Autodesk Fusion 360 part; units mm, degrees
(part 3 of 3)
  constraint equal A304 A396
  constraint tangent L88 A397
  constraint tangent L89 A397
  constraint equal A304 A397
  constraint tangent L88 A398
  constraint tangent L90 A398
  constraint equal A304 A398
  constraint tangent L90 A399
  constraint tangent L91 A399
  constraint equal A304 A399
  constraint tangent L93 A400
  constraint tangent L95 A400
  constraint equal A304 A400
  constraint tangent L92 A401
  constraint tangent L93 A401
  constraint equal A304 A401
  constraint tangent L92 A402
  constraint tangent L94 A402
  constraint equal A304 A402
  constraint tangent L94 A403
  constraint tangent L95 A403
  constraint equal A304 A403
  constraint tangent L120 A404
  constraint tangent L121 A404
  constraint equal A304 A404
  constraint tangent L120 A405
  constraint tangent L123 A405
  constraint equal A304 A405
  constraint tangent L166 A406
  constraint tangent L167 A406
  constraint equal A304 A406
  constraint tangent L165 A407
  constraint tangent L166 A407
  constraint equal A304 A407
  constraint tangent L164 A408
  constraint tangent L165 A408
  constraint equal A304 A408
  constraint tangent L160 A409
  constraint tangent L163 A409
  constraint equal A304 A409
  constraint tangent L162 A410
  constraint tangent L163 A410
  constraint equal A304 A410
  constraint tangent L161 A411
  constraint tangent L162 A411
  constraint equal A304 A411
  constraint tangent L160 A412
  constraint tangent L161 A412
  constraint equal A304 A412
  constraint tangent L432 A413
  constraint tangent L435 A413
  constraint equal A304 A413
  constraint tangent L434 A414
  constraint tangent L435 A414
  constraint equal A304 A414
  constraint tangent L405 A415
  constraint tangent L406 A415
  constraint equal A304 A415
  constraint tangent L404 A416
  constraint tangent L405 A416
  constraint equal A304 A416
  constraint tangent L404 A417
  constraint tangent L407 A417
  constraint equal A304 A417
  constraint tangent L406 A418
  constraint tangent L407 A418
  constraint equal A304 A418
  constraint tangent L401 A419
  constraint tangent L402 A419
  constraint equal A304 A419
  constraint tangent L400 A420
  constraint tangent L401 A420
  constraint equal A304 A420
  constraint tangent L400 A421
  constraint tangent L403 A421
  constraint equal A304 A421
  constraint tangent L402 A422
  constraint tangent L403 A422
  constraint equal A304 A422
  constraint tangent L158 A423
  constraint tangent L159 A423
  constraint equal A304 A423
  constraint tangent L156 A424
  constraint tangent L159 A424
  constraint equal A304 A424
  constraint tangent L156 A425
  constraint tangent L157 A425
  constraint equal A304 A425
  constraint tangent L157 A426
  constraint tangent L158 A426
  constraint equal A304 A426
  constraint tangent L116 A427
  constraint tangent L119 A427
  constraint equal A304 A427
  constraint tangent L117 A428
  constraint tangent L118 A428
  constraint equal A304 A428
  constraint tangent L116 A429
  constraint tangent L117 A429
  constraint equal A304 A429
  constraint tangent L112 A430
  constraint tangent L115 A430
  constraint equal A304 A430
  constraint tangent L114 A431
  constraint tangent L115 A431
  constraint equal A304 A431
  constraint tangent L113 A432
  constraint tangent L114 A432
  constraint equal A304 A432
  constraint tangent L112 A433
  constraint tangent L113 A433
  constraint equal A304 A433
  constraint tangent L108 A434
  constraint tangent L111 A434
  constraint equal A304 A434
  constraint tangent L110 A435
  constraint tangent L111 A435
  constraint equal A304 A435
  constraint tangent L109 A436
  constraint tangent L110 A436
  constraint equal A304 A436
  constraint tangent L108 A437
  constraint tangent L109 A437
  constraint equal A304 A437
  constraint tangent L152 A438
  constraint tangent L153 A438
  constraint equal A304 A438
  constraint tangent L153 A439
  constraint tangent L154 A439
  constraint equal A304 A439
  constraint tangent L154 A440
  constraint tangent L155 A440
  constraint equal A304 A440
  constraint tangent L152 A441
  constraint tangent L155 A441
  constraint equal A304 A441
  constraint tangent L105 A442
  constraint tangent L106 A442
  constraint equal A304 A442
  constraint tangent L104 A443
  constraint tangent L105 A443
  constraint equal A304 A443
  constraint tangent L104 A444
  constraint tangent L107 A444
  constraint equal A304 A444
  constraint tangent L106 A445
  constraint tangent L107 A445
  constraint equal A304 A445
  constraint tangent L41 A446
  constraint tangent L42 A446
  constraint equal A304 A446
  constraint tangent L40 A447
  constraint tangent L41 A447
  constraint equal A304 A447
  constraint tangent L396 A448
  constraint tangent L397 A448
  constraint equal A304 A448
  constraint tangent L397 A449
  constraint tangent L398 A449
  constraint equal A304 A449
  constraint tangent L46 A450
  constraint tangent L47 A450
  constraint equal A304 A450
  constraint tangent L45 A451
  constraint tangent L46 A451
  constraint equal A304 A451
  constraint tangent L44 A452
  constraint tangent L47 A452
  constraint equal A304 A452
  constraint tangent L44 A453
  constraint tangent L45 A453
  constraint equal A304 A453
  constraint tangent L42 A454
  constraint tangent L43 A454
  constraint equal A304 A454
  constraint tangent L40 A455
  constraint tangent L43 A455
  constraint equal A304 A455
  constraint tangent L392 A456
  constraint tangent L395 A456
  constraint equal A304 A456
  constraint tangent L392 A457
  constraint tangent L393 A457
  constraint equal A304 A457
  constraint tangent L393 A458
  constraint tangent L394 A458
  constraint equal A304 A458
  constraint tangent L394 A459
  constraint tangent L395 A459
  constraint equal A304 A459
  constraint tangent L398 A460
  constraint tangent L399 A460
  constraint equal A304 A460
  constraint tangent L396 A461
  constraint tangent L399 A461
  constraint equal A304 A461
  constraint tangent L436 A462
  constraint tangent L439 A462
  constraint tangent L436 A463
  constraint tangent L437 A463
  constraint tangent L437 A464
  constraint tangent L438 A464
  constraint equal A463 A464
  constraint tangent L438 A465
  constraint tangent L439 A465
  constraint equal A463 A465
  constraint tangent L440 A466
  constraint tangent L441 A466
  constraint equal A463 A466
  constraint tangent L440 A467
  constraint tangent L443 A467
  constraint equal A463 A467
  constraint tangent L442 A468
  constraint tangent L443 A468
  constraint equal A463 A468
  constraint tangent L441 A469
  constraint tangent L442 A469
  constraint equal A463 A469
  constraint tangent L447 A470
  constraint tangent L448 A470
  constraint equal A463 A470
  constraint tangent L450 A471
  constraint tangent L451 A471
  constraint equal A463 A471
  constraint tangent L446 A472
  constraint tangent L448 A472
  constraint equal A463 A472
  constraint tangent L451 A473
  constraint tangent L452 A473
  constraint equal A463 A473
  constraint tangent L449 A474
  constraint tangent L450 A474
  constraint equal A463 A474
  constraint tangent L445 A475
  constraint tangent L447 A475
  constraint equal A463 A475
  constraint tangent L449 A476
  constraint tangent L452 A476
  constraint equal A463 A476
  constraint tangent L445 A477
  constraint tangent L446 A477
  constraint equal A463 A477
  measures "d35" diameter of A8
  measures "d36" radius of A9
  measures "d37" radius of A10
  measures "d38" radius of A11
  measures "d40" radius of A12
  measures "d41" radius of A13
  measures "d42" diameter of A14
  measures "d43" distance of L0.start L0.end
  measures "d44" diameter of A3
  measures "d45" diameter of A2
  measures "d46" diameter of A4
  measures "d47" diameter of A18
  measures "d48" diameter of A28
  measures "d49" distance of A18.centre L16.start
  measures "d50" distance of L16.start L16.end
  measures "d51" diameter of A15
  measures "d52" diameter of A19
  measures "d53" distance of L16.start L17.end
  measures "d54" diameter of A21
  measures "d55" diameter of A20
  measures "d59" radius of A16
  measures "d60" diameter of A17
  measures "d61" diameter of A29
  measures "d62" diameter of A27
  measures "d63" angle of L21 L22
  measures "d64" diameter of A24
  measures "d65" diameter of A25
  measures "d66" radius of A26
  measures "d67" radius of A44
  measures "d68" radius of A45
  measures "d69" diameter of A46
  measures "d70" diameter of A47
  measures "d72" distance of L27 L28
  measures "d73" diameter of A50
  measures "d74" diameter of A48
  measures "d75" diameter of A49
  measures "d176" radius of A69
  measures "d177" radius of A304
  measures "d178" radius of A462
  measures "d179" radius of A463
sketch "Sketch7" plane through (0, 0, 0) normal (0, 0, 1) x (1, 0, 0)
sketch "Sketch5" plane through (0, 0, 0) normal (0, 0, 1) x (1, 0, 0)
  line L0 (684, -14) -> (688, -14)
  line L1 (688, -14) -> (688, -23)
  line L2 (688, -23) -> (684, -23)
  line L3 (684, -23) -> (684, -14)
  constraint horizontal L0
  constraint vertical L1
  constraint horizontal L2
  constraint vertical L3
sketch "Sketch4" plane through (0, 0, 0) normal (0, 0, 1) x (1, 0, 0)
sketch "Sketch3" plane through (0, 0, 0) normal (0, 0, 1) x (1, 0, 0)
sketch "Sketch6" plane through (0, 0, 0) normal (0, 0, 1) x (1, 0, 0)
sketch "Sketch8" plane through (0, 0, 0) normal (0, 0, 1) x (1, 0, 0)
extrude "Extrude1" add sketch "Sketch2" along normal blind 10 contours L440 L441 L442 L443 A466 A467 A468 A469
extrude "Extrude2" add sketch "Sketch2" along normal blind 14 contours L196 L197 L198 L199 A304 A305 A306 A307 | L200 L201 L202 L203 A308 A309 A310 A311 | L204 L205 L206 L207 A312 A313 A314 A315
equation "d145 = 'Ecs'"
equation "d147 = 'F1'"
equation "d149 = 'F2'"
equation "d151 = 'F3'"
equation "d153 = 'F4'"
equation "d155 = 'F5'"
equation "d157 = 'F6'"
equation "d159 = 'F7'"
equation "d161 = 'F8'"
equation "d163 = 'F9'"
equation "d165 = 'F10'"
equation "d167 = 'F11'"
equation "d169 = 'F12'"
equation "d173 = 'delete'"
equation "d175 = 'delete'"
